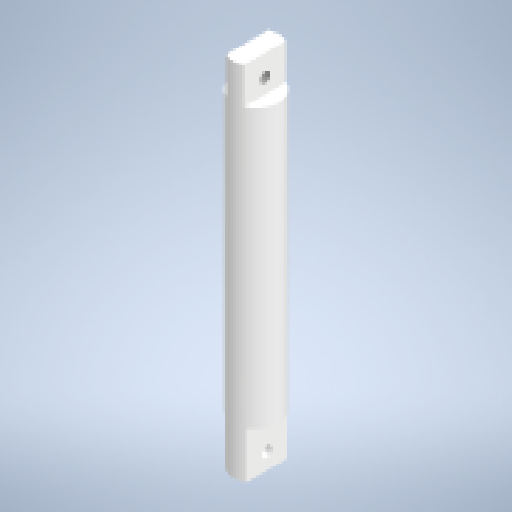
# Autodesk Inventor part: extensio
Saved by Autodesk Inventor 2024.3 (Build 283343000, 343)
## iProperties
Created: 2024-05-08
Part Number: extensio
Material: Tuberías de PVC
Document SubType Name: Modeling
Designer: riera
Density: 1.4 g/cm^3
Appearance: Suave - Blanco
Author: riera
Autodesk Inventor part; units mm, degrees
ref_plane "YZ Plane" through (0, 0, 0) normal (1, 0, 0) x (0, 1, 0)
ref_plane "XZ Plane" through (0, 0, 0) normal (0, 1, 0) x (-1, 0, 0)
ref_plane "XY Plane" through (0, 0, 0) normal (0, 0, 1) x (1, 0, 0)
sketch "Boceto1" plane through (0, 0, 0) normal (0, 1, 0) x (-1, 0, 0)
  circle A0 centre (0, 0) radius 6.375
  dimension "d0" = 12.75
  constraints: 1 centre point, 1 coincident
  measures "d0" diameter of A0
extrude "Extrusión1" add sketch "Boceto1" along normal blind 100
sketch "Boceto2" plane through (0, 100, 0) normal (0, 1, 0) x (1, 0, 0)
  line L0 (2.5, 5.8644) -> (2.5, -5.8644)
  line L1 (-2.5, -5.8644) -> (-2.5, 5.8644)
  arc A0 (-2.5, 5.8644) -> (-2.5, -5.8644) centre (0, 0) ccw
  arc A1 (2.5, -5.8644) -> (2.5, 5.8644) centre (0, 0) ccw
  point P0 (2.5, 0)
  point P1 (-2.5, 0)
  dimension "d5" = 5
  dimension "d6" = 6.375
  dimension "d7" = 6.375
  dimension "d8" = 11.7287
  constraints: 4 end point, 4 point on circle, 2 centre point, 2 horizontal alignment, 2 midpoint, 1 coincident, 1 parallel
  measures "d5" distance between parallel lines of L0 L1
  measures "d6" radius of A1
  measures "d7" radius of A0
  measures "d8" distance of L1.start L1.end
extrude "Extrusión2" cut sketch "Boceto2" against normal blind 10
sketch "Boceto3" plane through (-2.5, 100, -5.8644) normal (-1, 0, 0) x (0, 0, 1)
  circle A0 centre (5.8644, -6) radius 1.5
  line L0 (0, -10) -> (11.7287, -10) projected
  line L1 (0, -10) -> (11.7287, -10) projected
  point P0 (5.8644, -100)
  point P1 (5.8644, -10)
  point P2 (5.8644, -10)
  dimension "d11" = 3
  dimension "d12" = 4
  constraints: 2 midpoint, 1 centre point, 1 vertical alignment
  measures "d11" diameter of A0
  measures "d12" distance of point (5.864, -10) A0.centre
extrude "Extrusión3" cut sketch "Boceto3" against normal through all
sketch "Boceto5" plane through (0, 0, 0) normal (0, -1, 0) x (1, 0, 0)
  line L0 (3, 5.625) -> (3, -5.625)
  line L1 (-3, -5.625) -> (-3, 5.625)
  arc A0 (-3, 5.625) -> (-3, -5.625) centre (0, 0) ccw
  arc A1 (3, -5.625) -> (3, 5.625) centre (0, 0) ccw
  point P0 (3, 0)
  constraints: 4 end point, 4 point on circle, 2 centre point, 1 coincident, 1 horizontal alignment, 1 midpoint, 1 parallel
extrude "Extrusión5" cut sketch "Boceto5" against normal blind 13
sketch "Boceto6" plane through (3, 0, 5.625) normal (1, 0, 0) x (0, 0, -1)
  circle A0 centre (5.625, 4.5) radius 1.5
  line L0 (11.25, 0) -> (0, 0) projected
  point P0 (5.625, 0)
  point P1 (5.625, 0)
  point P2 (5.625, 0)
  dimension "d26" = 3
  dimension "d27" = 4.5
  constraints: 2 midpoint, 1 centre point, 1 vertical alignment
  measures "d26" diameter of A0
  measures "d27" distance of point (5.625, 0) A0.centre
extrude "Extrusión6" cut sketch "Boceto6" against normal through all
thread "Rosca1" size "M3x0.5" class "6H" standard "ANSI Metric M Profile" full length
scale "Escala1" factors (0.8, 0.8, 0.8) then translate (0, 10, 0) bodies 1
